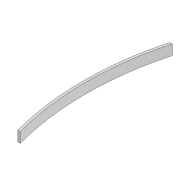
# Autodesk Inventor part: Support_strip
Saved by Autodesk Inventor 2022 (Build 260153000, 153)
## iProperties
Created: 2022-07-27
Part Number: Support_strip
Material: Generic
Document SubType Name: Modeling
Designer: dell
Density: 1 g/cm^3
Appearance: Default
Author: dell
Autodesk Inventor part; units mm, degrees
ref_plane "YZ Plane" through (0, 0, 0) normal (1, 0, 0) x (0, 1, 0)
ref_plane "XZ Plane" through (0, 0, 0) normal (0, 1, 0) x (-1, 0, 0)
ref_plane "XY Plane" through (0, 0, 0) normal (0, 0, 1) x (1, 0, 0)
sketch "Sketch1" plane through (0, 0, 0) normal (0, 1, 0) x (-1, 0, 0)
  arc A0 (0, -30) -> (0, 0) centre (-55.25, -15) ccw
  line L0 (0, 0) -> (0, -30) construction
  line L1 (0, -30) -> (2, -30) construction
  line L2 (2, -30) -> (2, 0) construction
  line L3 (2, 0) -> (0, 0) construction
  line L4 (0, 0) -> (0.5, 0)
  line L5 (0, -30) -> (0.5, -30)
  arc A1 (0.5, -30) -> (0.5, 0) centre (-55.0044, -15) ccw
  dimension "d0" = 30
  dimension "d1" = 2
  dimension "d4" = 0.5
  dimension "d5" = 0.5
  constraints: 12 end point, 4 point on circle, 2 centre point, 2 parallel, 2 point on line, 2 tangent, 1 perpendicular, 1 vertical
  measures "d0" distance of L0.start L0.end
  measures "d1" distance of L1.end L0.end
  measures "d4" distance of L0.end L5.end
  measures "d5" distance of L0.start L4.end
extrude "Extrusion1" add sketch "Sketch1" along normal blind 2
body "Solid1"
